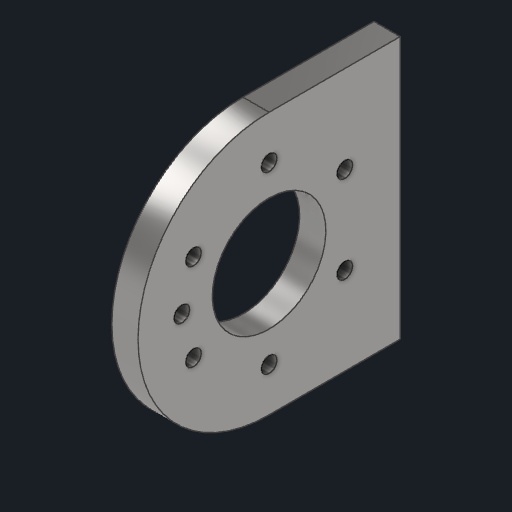
# Autodesk Inventor part: SYSTEM-FLANGE-K60
Saved by Autodesk Inventor 2025.3 (Build 293356030, 356C)
## iProperties
Created: 2025-11-27
Part Number: SYSTEM-FLANGE-K60
Material: Aluminum 6061
Document SubType Name: Modeling
Designer: lstk1ng
Density: 2.7 g/cm^3
Appearance: Semi-Polished
Mass: 661.045 g
Surface Area: 467.104 cm^2
Volume: 244.832 cm^3
Author: lstk1ng
Autodesk Inventor part; units mm, degrees
ref_plane "YZ Plane" through (0, 0, 0) normal (1, 0, 0) x (0, 1, 0)
ref_plane "XZ Plane" through (0, 0, 0) normal (0, 1, 0) x (-1, 0, 0)
ref_plane "XY Plane" through (0, 0, 0) normal (0, 0, 1) x (1, 0, 0)
sketch "Sketch1" plane through (0, 0, 0) normal (1, 0, 0) x (0, 1, 0)
  circle A0 centre (0, 0) radius 62.5 construction
  circle A1 centre (0, 0) radius 50 construction
  circle A2 centre (0, 50) radius 4.5
  line L0 (0, 0) -> (25, 43.3013) construction
  line L1 (0, 0) -> (50, 0) construction
  circle A3 centre (25, 43.3013) radius 4.5
  circle A4 centre (-25, 43.3013) radius 4.5
  circle A5 centre (-50, 0) radius 4.5
  circle A6 centre (-25, -43.3013) radius 4.5
  circle A7 centre (25, -43.3013) radius 4.5
  circle A8 centre (50, 0) radius 4.5
  circle A9 centre (0, 0) radius 32.5
  arc A10 (75, 0) -> (-75, 0) centre (0, 0) ccw
  line L2 (-75, 0) -> (-75, -75)
  line L3 (-75, -75) -> (0, -75)
  line L4 (0, -75) -> (75, -75)
  line L5 (75, -75) -> (75, 0)
  dimension "d0" = 125
  dimension "d1" = 100
  dimension "d2" = 9
  dimension "d3" = 60
  dimension "d4" = 9
  dimension "d7" = 360
  dimension "d9" = 65
  dimension "d10" = 150
  constraints: 12 end point, 11 centre point, 5 coincident, 4 point on circle, 4 tangent, 1 equal length, 1 horizontal, 1 point on line, 1 vertical, 13 other
  measures "d0" diameter of A0
  measures "d1" diameter of A1
  measures "d2" diameter of A2
  measures "d3" angle of L1 L0
  measures "d4" diameter of A3
  measures "d9" diameter of A9
  measures "d10" diameter of A10
extrude "Extrusion1" add sketch "Sketch1" along normal blind 15
body "Solid1"
